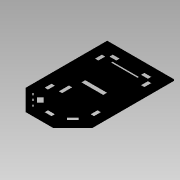
# Autodesk Inventor part: Base Kepala
Saved by Autodesk Inventor 2015 SP1 (Build 190203100, 203)
## iProperties
Created: 2015-02-13
Part Number: Base Kepala
Material: Generic
Document SubType Name: Modeling
Designer: Rafi Kurnia Putra
Density: 1 g/cm^3
Appearance: Default(1)
Author: Rafi Kurnia Putra
Autodesk Inventor part; units mm, degrees
ref_plane "YZ Plane" through (0, 0, 0) normal (1, 0, 0) x (0, 1, 0)
ref_plane "XZ Plane" through (0, 0, 0) normal (0, 1, 0) x (-1, 0, 0)
ref_plane "XY Plane" through (0, 0, 0) normal (0, 0, 1) x (1, 0, 0)
sketch "Sketch1" plane through (0, 0, 0) normal (0, 1, 0) x (-1, 0, 0)
  line L0 (31.6823, -78.8894) -> (44.0567, -66.5151)
  line L1 (24.6113, -71.8184) -> (31.6823, -78.8894)
  line L2 (36.9856, -59.444) -> (24.6113, -71.8184)
  line L3 (44.0567, -66.5151) -> (36.9856, -59.444)
  line L4 (8.75, -88.3884) -> (8.75, -78.3884)
  line L5 (-8.75, -88.3884) -> (8.75, -88.3884)
  line L6 (8.75, -78.3884) -> (-8.75, -78.3884)
  line L7 (-8.75, -78.3884) -> (-8.75, -88.3884)
  line L8 (-31.6827, -78.8894) -> (-24.6116, -71.8184)
  line L9 (-24.6116, -71.8184) -> (-36.986, -59.444)
  line L10 (-44.057, -66.5151) -> (-31.6827, -78.8894)
  line L11 (-36.986, -59.444) -> (-44.057, -66.5151)
  line L12 (-53.5557, -43.5826) -> (-43.5557, -43.5826)
  line L13 (-43.5557, -43.5826) -> (-43.5557, -26.0826)
  line L14 (-43.5557, -26.0826) -> (-53.5557, -26.0826)
  line L15 (-53.5557, -26.0826) -> (-53.5557, -43.5826)
  line L16 (-53.556, 80.1674) -> (-53.556, 62.6674)
  line L17 (-43.556, 80.1674) -> (-53.556, 80.1674)
  line L18 (-43.556, 62.6674) -> (-43.556, 80.1674)
  line L19 (-53.556, 62.6674) -> (-43.556, 62.6674)
  line L20 (-42.0848, 91.6386) -> (-42.0848, 81.6386)
  line L21 (-42.0848, 81.6386) -> (-24.5848, 81.6386)
  line L22 (-24.5848, 81.6386) -> (-24.5848, 91.6386)
  line L23 (-24.5848, 91.6386) -> (-42.0848, 91.6386)
  line L24 (42.0848, 91.6386) -> (24.5848, 91.6386)
  line L25 (42.0848, 81.6386) -> (42.0848, 91.6386)
  line L26 (24.5848, 81.6386) -> (42.0848, 81.6386)
  line L27 (24.5848, 91.6386) -> (24.5848, 81.6386)
  line L28 (43.556, 80.1674) -> (43.556, 62.6674)
  line L29 (53.556, 80.1674) -> (43.556, 80.1674)
  line L30 (53.556, 62.6674) -> (53.556, 80.1674)
  line L31 (43.556, 62.6674) -> (53.556, 62.6674)
  circle A0 centre (37.593, 75.6756) radius 1.75
  circle A1 centre (32.8575, 75.4371) radius 1.75
  circle A2 centre (50.5965, 88.6786) radius 1.75
  line L32 (29.3575, 78.4256) -> (-29.3575, 78.4256)
  line L33 (29.3575, 72.4486) -> (29.3575, 78.4256)
  line L34 (-29.3575, 72.4486) -> (29.3575, 72.4486)
  line L35 (-29.3575, 78.4256) -> (-29.3575, 72.4486)
  circle A3 centre (-32.8575, 75.4371) radius 1.75
  circle A4 centre (-37.593, 75.6756) radius 1.75
  circle A5 centre (-50.5965, 88.6786) radius 1.75
  line L36 (-24.5, 4.9331) -> (24.5, 4.9331)
  circle A6 centre (28, 4.9331) radius 1.75
  circle A7 centre (32.442, 26.7171) radius 1.5
  circle A8 centre (38, 31.4596) radius 1.75
  circle A9 centre (50.5965, 18.9376) radius 1.75
  circle A10 centre (32.4485, 53.6756) radius 1.75
  circle A11 centre (-32.4355, 53.6756) radius 1.75
  circle A12 centre (-50.5965, 18.9376) radius 1.75
  circle A13 centre (-32.442, 26.7171) radius 1.5
  circle A14 centre (-28, 4.9331) radius 1.75
  line L37 (-22.2, -10.9442) -> (-32, -10.9442)
  line L38 (-22.2, -35.1896) -> (-22.2, -10.9442)
  line L39 (-32, -35.1896) -> (-22.2, -35.1896)
  line L40 (-32, -10.9442) -> (-32, -35.1896)
  circle A15 centre (-49.906, -55.5042) radius 1.75
  circle A16 centre (-37.593, -48.9392) radius 1.75
  circle A17 centre (-20, -65.0669) radius 1.75
  circle A18 centre (13.2193, -19.3896) radius 1.75
  circle A19 centre (13.2193, -43.7996) radius 1.75
  circle A20 centre (20, -65.0669) radius 1.75
  circle A21 centre (37.593, -48.9392) radius 1.75
  circle A22 centre (39.7053, -43.7996) radius 1.75
  circle A23 centre (39.7053, -19.3896) radius 1.75
  circle A24 centre (49.9057, -55.5042) radius 1.75
  line L41 (43.5557, -43.5826) -> (53.5557, -43.5826)
  line L42 (43.5557, -26.0826) -> (43.5557, -43.5826)
  line L43 (53.5557, -26.0826) -> (43.5557, -26.0826)
  line L44 (53.5557, -43.5826) -> (53.5557, -26.0826)
  line L45 (24.5, 4.9331) -> (24.5, 15.9376)
  line L46 (24.5, 15.9376) -> (-24.5, 15.9376)
  line L47 (-24.5, 15.9376) -> (-24.5, 4.9331)
  circle A25 centre (14, 31.4596) radius 1.75
  circle A26 centre (-27.94, -53.8096) radius 1.75
  circle A27 centre (20.32, -47.4596) radius 1.75
  line L48 (70.4053, -63.9933) -> (29.1627, -105.2363)
  line L49 (29.1627, -105.2363) -> (-29.1634, -105.2362)
  line L50 (-29.1634, -105.2362) -> (-70.4063, -63.9936)
  line L51 (-70.4063, -63.9936) -> (-70.4063, 108.2408)
  line L52 (-70.4063, 108.2408) -> (70.4053, 108.2411)
  line L53 (70.4053, 108.2411) -> (70.4053, -63.9933)
  line L54 (37.7622, -79.6663) -> (44.8333, -72.5952)
  line L55 (44.8333, -72.5952) -> (46.2475, -74.0094)
  line L56 (46.2475, -74.0094) -> (39.1764, -81.0805)
  line L57 (39.1764, -81.0805) -> (37.7622, -79.6663)
  line L58 (37.7622, -79.6663) -> (46.2475, -74.0094) construction
  line L59 (44.8333, -72.5952) -> (39.1764, -81.0805) construction
  line L60 (34.2266, -83.2018) -> (27.1556, -90.2729)
  line L61 (27.1556, -90.2729) -> (28.5698, -91.6871)
  line L62 (28.5698, -91.6871) -> (35.6409, -84.616)
  line L63 (35.6409, -84.616) -> (34.2266, -83.2018)
  line L64 (34.2266, -83.2018) -> (28.5698, -91.6871) construction
  line L65 (27.1556, -90.2729) -> (35.6409, -84.616) construction
  line L66 (55.4401, -61.9888) -> (48.369, -69.0599)
  line L67 (48.369, -69.0599) -> (49.7828, -70.4737)
  line L68 (49.7828, -70.4737) -> (56.8539, -63.4026)
  line L69 (56.8539, -63.4026) -> (55.4401, -61.9888)
  line L70 (55.4401, -61.9888) -> (49.7828, -70.4737) construction
  line L71 (48.369, -69.0599) -> (56.8539, -63.4026) construction
  line L72 (5, -93.2363) -> (15, -93.2363) construction
  line L73 (-10, -93.2363) -> (-20, -93.2363)
  line L74 (-20, -93.2363) -> (-20, -95.2363)
  line L75 (-20, -95.2363) -> (-10, -95.2363)
  line L76 (-10, -95.2363) -> (-10, -93.2363)
  line L77 (-10, -93.2363) -> (-20, -95.2363) construction
  line L78 (-20, -93.2363) -> (-10, -95.2363) construction
  line L79 (-10, -93.2363) -> (0, -93.2363) construction
  line L80 (20, -95.2363) -> (10, -95.2363)
  line L81 (10, -95.2363) -> (10, -93.237)
  line L82 (10, -93.237) -> (20, -93.237)
  line L83 (20, -93.237) -> (20, -95.2363)
  line L84 (20, -95.2363) -> (10, -93.237) construction
  line L85 (10, -95.2363) -> (20, -93.237) construction
  line L86 (-7.5214, 96.2408) -> (7.4786, 96.2408)
  line L87 (7.4786, 96.2408) -> (7.4786, 98.2408)
  line L88 (7.4786, 98.2408) -> (-7.5214, 98.2408)
  line L89 (-7.5214, 98.2408) -> (-7.5214, 96.2408)
  line L90 (-7.5214, 96.2408) -> (7.4786, 98.2408) construction
  line L91 (7.4786, 96.2408) -> (-7.5214, 98.2408) construction
  line L92 (-7.5214, 96.2408) -> (7.4786, 96.2408) construction
  line L93 (60.4053, 25.443) -> (60.4053, 10.443)
  line L94 (60.4053, 10.443) -> (58.4053, 10.443)
  line L95 (58.4053, 10.443) -> (58.4053, 25.443)
  line L96 (58.4053, 25.443) -> (60.4053, 25.443)
  line L97 (60.4053, 25.443) -> (58.4053, 10.443) construction
  line L98 (60.4053, 10.443) -> (58.4053, 25.443) construction
  line L99 (-37.8487, -79.5805) -> (-44.9198, -72.5095)
  line L100 (-44.9198, -72.5095) -> (-46.334, -73.9237)
  line L101 (-46.334, -73.9237) -> (-39.2629, -80.9947)
  line L102 (-39.2629, -80.9947) -> (-37.8487, -79.5805)
  line L103 (-37.8487, -79.5805) -> (-46.334, -73.9237) construction
  line L104 (-34.3131, -83.116) -> (-27.242, -90.1871)
  line L105 (-27.242, -90.1871) -> (-28.6562, -91.6013)
  line L106 (-28.6562, -91.6013) -> (-35.7273, -84.5302)
  line L107 (-35.7273, -84.5302) -> (-34.3131, -83.116)
  line L108 (-34.3131, -83.116) -> (-28.6562, -91.6013) construction
  line L109 (-27.242, -90.1871) -> (-35.7273, -84.5302) construction
  line L110 (-55.5071, -61.8836) -> (-48.4359, -68.9546)
  line L111 (-48.4359, -68.9546) -> (-49.8695, -70.3882)
  line L112 (-49.8695, -70.3882) -> (-56.9406, -63.3172)
  line L113 (-56.9406, -63.3172) -> (-55.5071, -61.8836)
  line L114 (-55.5071, -61.8836) -> (-49.8695, -70.3882) construction
  line L115 (-48.4359, -68.9546) -> (-56.9406, -63.3172) construction
  line L116 (-60.4053, 25.443) -> (-60.4053, 10.443)
  line L117 (-60.4053, 10.443) -> (-58.4053, 10.443)
  line L118 (-58.4053, 10.443) -> (-58.4053, 25.443)
  line L119 (-58.4053, 25.443) -> (-60.4053, 25.443)
  line L120 (-60.4053, 25.443) -> (-58.4053, 10.443) construction
  line L121 (-60.4053, 10.443) -> (-58.4053, 25.443) construction
  line L122 (-58.4053, 42.943) -> (-58.4053, 57.943)
  line L123 (-58.4053, 57.943) -> (-60.4053, 57.943)
  line L124 (-60.4053, 57.943) -> (-60.4053, 42.943)
  line L125 (-60.4053, 57.943) -> (-58.4053, 42.943) construction
  line L126 (-60.4053, 42.943) -> (-58.4053, 57.943) construction
  line L127 (-60.4053, 42.943) -> (-58.4053, 42.943)
  line L128 (-58.4053, 75.443) -> (-58.4053, 90.443)
  line L129 (-58.4053, 90.443) -> (-60.4053, 90.443)
  line L130 (-60.4053, 90.443) -> (-60.4053, 75.443)
  line L131 (-60.4053, 90.443) -> (-58.4053, 75.443) construction
  line L132 (-60.4053, 75.443) -> (-58.4053, 90.443) construction
  line L133 (-60.4053, 75.443) -> (-58.4053, 75.443)
  line L134 (-58.4053, -22.057) -> (-58.4053, -7.057)
  line L135 (-58.4053, -7.057) -> (-60.4053, -7.057)
  line L136 (-60.4053, -7.057) -> (-60.4053, -22.057)
  line L137 (-60.4053, -7.057) -> (-58.4053, -22.057) construction
  line L138 (-60.4053, -22.057) -> (-58.4053, -7.057) construction
  line L139 (-60.4053, -22.057) -> (-58.4053, -22.057)
  line L140 (-58.4053, 10.443) -> (-58.4053, 25.443)
  line L141 (-58.4053, 25.443) -> (-60.4053, 25.443)
  line L142 (-60.4053, 25.443) -> (-60.4053, 10.443)
  line L143 (-60.4053, 25.443) -> (-58.4053, 10.443) construction
  line L144 (-60.4053, 10.443) -> (-58.4053, 25.443) construction
  line L145 (-60.4053, 10.443) -> (-58.4053, 10.443)
  line L146 (-58.4053, 42.943) -> (-58.4053, 57.943)
  line L147 (-58.4053, 57.943) -> (-60.4053, 57.943)
  line L148 (-60.4053, 57.943) -> (-60.4053, 42.943)
  line L149 (-60.4053, 57.943) -> (-58.4053, 42.943) construction
  line L150 (-60.4053, 42.943) -> (-58.4053, 57.943) construction
  line L151 (-60.4053, 42.943) -> (-58.4053, 42.943)
  line L152 (-58.4063, -54.3943) -> (-58.4063, -39.3943)
  line L153 (-58.4063, -39.3943) -> (-60.4063, -39.3943)
  line L154 (-60.4063, -39.3943) -> (-60.4063, -54.3943)
  line L155 (-60.4063, -39.3943) -> (-58.4063, -54.3943) construction
  line L156 (-60.4063, -54.3943) -> (-58.4063, -39.3943) construction
  line L157 (-60.4063, -54.3943) -> (-58.4063, -54.3943)
  line L158 (-58.4063, -21.8943) -> (-58.4063, -6.8943)
  line L159 (-58.4063, -6.8943) -> (-60.4063, -6.8943)
  line L160 (-60.4063, -6.8943) -> (-60.4063, -21.8943)
  line L161 (-60.4063, -6.8943) -> (-58.4063, -21.8943) construction
  line L162 (-60.4063, -21.8943) -> (-58.4063, -6.8943) construction
  line L163 (-60.4063, -21.8943) -> (-58.4063, -21.8943)
  line L164 (-58.4053, 10.443) -> (-58.4053, 25.443)
  line L165 (-58.4053, 25.443) -> (-60.4053, 25.443)
  line L166 (-60.4053, 25.443) -> (-60.4053, 10.443)
  line L167 (-60.4053, 25.443) -> (-58.4053, 10.443) construction
  line L168 (-60.4053, 10.443) -> (-58.4053, 25.443) construction
  line L169 (-60.4053, 10.443) -> (-58.4053, 10.443)
  line L170 (15.4786, 96.2409) -> (30.4786, 96.2409)
  line L171 (30.4786, 96.2409) -> (30.4786, 98.2409)
  line L172 (30.4786, 98.2409) -> (15.4786, 98.2409)
  line L173 (15.4786, 98.2409) -> (15.4786, 96.2409)
  line L174 (15.4786, 96.2409) -> (30.4786, 98.2409) construction
  line L175 (30.4786, 96.2409) -> (15.4786, 98.2409) construction
  line L176 (15.4786, 96.2409) -> (30.4786, 96.2409) construction
  line L177 (38.4786, 96.2409) -> (53.4786, 96.2409)
  line L178 (53.4786, 96.2409) -> (53.4786, 98.2409)
  line L179 (53.4786, 98.2409) -> (38.4786, 98.2409)
  line L180 (38.4786, 98.2409) -> (38.4786, 96.2409)
  line L181 (38.4786, 96.2409) -> (53.4786, 98.2409) construction
  line L182 (53.4786, 96.2409) -> (38.4786, 98.2409) construction
  line L183 (38.4786, 96.2409) -> (53.4786, 96.2409) construction
  line L184 (-30.5214, 96.2408) -> (-15.5214, 96.2408)
  line L185 (-15.5214, 96.2408) -> (-15.5214, 98.2408)
  line L186 (-15.5214, 98.2408) -> (-30.5214, 98.2408)
  line L187 (-30.5214, 98.2408) -> (-30.5214, 96.2408)
  line L188 (-30.5214, 96.2408) -> (-15.5214, 98.2408) construction
  line L189 (-15.5214, 96.2408) -> (-30.5214, 98.2408) construction
  line L190 (-30.5214, 96.2408) -> (-15.5214, 96.2408) construction
  line L191 (-7.5214, 96.2408) -> (7.4786, 96.2408)
  line L192 (7.4786, 96.2408) -> (7.4786, 98.2408)
  line L193 (7.4786, 98.2408) -> (-7.5214, 98.2408)
  line L194 (-7.5214, 98.2408) -> (-7.5214, 96.2408)
  line L195 (-7.5214, 96.2408) -> (7.4786, 98.2408) construction
  line L196 (7.4786, 96.2408) -> (-7.5214, 98.2408) construction
  line L197 (-7.5214, 96.2408) -> (7.4786, 96.2408) construction
  line L198 (15.4786, 96.2409) -> (30.4786, 96.2409)
  line L199 (30.4786, 96.2409) -> (30.4786, 98.2409)
  line L200 (30.4786, 98.2409) -> (15.4786, 98.2409)
  line L201 (15.4786, 98.2409) -> (15.4786, 96.2409)
  line L202 (15.4786, 96.2409) -> (30.4786, 98.2409) construction
  line L203 (30.4786, 96.2409) -> (15.4786, 98.2409) construction
  line L204 (15.4786, 96.2409) -> (30.4786, 96.2409) construction
  line L205 (-53.5214, 96.2407) -> (-38.5214, 96.2407)
  line L206 (-38.5214, 96.2407) -> (-38.5214, 98.2407)
  line L207 (-38.5214, 98.2407) -> (-53.5214, 98.2407)
  line L208 (-53.5214, 98.2407) -> (-53.5214, 96.2407)
  line L209 (-53.5214, 96.2407) -> (-38.5214, 98.2407) construction
  line L210 (-38.5214, 96.2407) -> (-53.5214, 98.2407) construction
  line L211 (-53.5214, 96.2407) -> (-38.5214, 96.2407) construction
  line L212 (-30.5214, 96.2408) -> (-15.5214, 96.2408)
  line L213 (-15.5214, 96.2408) -> (-15.5214, 98.2408)
  line L214 (-15.5214, 98.2408) -> (-30.5214, 98.2408)
  line L215 (-30.5214, 98.2408) -> (-30.5214, 96.2408)
  line L216 (-30.5214, 96.2408) -> (-15.5214, 98.2408) construction
  line L217 (-15.5214, 96.2408) -> (-30.5214, 98.2408) construction
  line L218 (-30.5214, 96.2408) -> (-15.5214, 96.2408) construction
  line L219 (-7.5214, 96.2408) -> (7.4786, 96.2408)
  line L220 (7.4786, 96.2408) -> (7.4786, 98.2408)
  line L221 (7.4786, 98.2408) -> (-7.5214, 98.2408)
  line L222 (-7.5214, 98.2408) -> (-7.5214, 96.2408)
  line L223 (-7.5214, 96.2408) -> (7.4786, 98.2408) construction
  line L224 (7.4786, 96.2408) -> (-7.5214, 98.2408) construction
  line L225 (-7.5214, 96.2408) -> (7.4786, 96.2408) construction
  line L226 (60.4053, 57.943) -> (60.4053, 42.943)
  line L227 (60.4053, 42.943) -> (58.4053, 42.943)
  line L228 (58.4053, 42.943) -> (58.4053, 57.943)
  line L229 (58.4053, 57.943) -> (60.4053, 57.943)
  line L230 (60.4053, 57.943) -> (58.4053, 42.943) construction
  line L231 (60.4053, 42.943) -> (58.4053, 57.943) construction
  line L232 (60.4053, 90.443) -> (60.4053, 75.443)
  line L233 (60.4053, 75.443) -> (58.4053, 75.443)
  line L234 (58.4053, 75.443) -> (58.4053, 90.443)
  line L235 (58.4053, 90.443) -> (60.4053, 90.443)
  line L236 (60.4053, 90.443) -> (58.4053, 75.443) construction
  line L237 (60.4053, 75.443) -> (58.4053, 90.443) construction
  line L238 (60.4053, -7.057) -> (60.4053, -22.057)
  line L239 (60.4053, -22.057) -> (58.4053, -22.057)
  line L240 (58.4053, -22.057) -> (58.4053, -7.057)
  line L241 (58.4053, -7.057) -> (60.4053, -7.057)
  line L242 (60.4053, -7.057) -> (58.4053, -22.057) construction
  line L243 (60.4053, -22.057) -> (58.4053, -7.057) construction
  line L244 (60.4053, 25.443) -> (60.4053, 10.443)
  line L245 (60.4053, 10.443) -> (58.4053, 10.443)
  line L246 (58.4053, 10.443) -> (58.4053, 25.443)
  line L247 (58.4053, 25.443) -> (60.4053, 25.443)
  line L248 (60.4053, 25.443) -> (58.4053, 10.443) construction
  line L249 (60.4053, 10.443) -> (58.4053, 25.443) construction
  line L250 (60.4053, 57.943) -> (60.4053, 42.943)
  line L251 (60.4053, 42.943) -> (58.4053, 42.943)
  line L252 (58.4053, 42.943) -> (58.4053, 57.943)
  line L253 (58.4053, 57.943) -> (60.4053, 57.943)
  line L254 (60.4053, 57.943) -> (58.4053, 42.943) construction
  line L255 (60.4053, 42.943) -> (58.4053, 57.943) construction
  line L256 (60.4053, -39.557) -> (60.4053, -54.557)
  line L257 (60.4053, -54.557) -> (58.4053, -54.557)
  line L258 (58.4053, -54.557) -> (58.4053, -39.557)
  line L259 (58.4053, -39.557) -> (60.4053, -39.557)
  line L260 (60.4053, -39.557) -> (58.4053, -54.557) construction
  line L261 (60.4053, -54.557) -> (58.4053, -39.557) construction
  line L262 (60.4053, -7.057) -> (60.4053, -22.057)
  line L263 (60.4053, -22.057) -> (58.4053, -22.057)
  line L264 (58.4053, -22.057) -> (58.4053, -7.057)
  line L265 (58.4053, -7.057) -> (60.4053, -7.057)
  line L266 (60.4053, -7.057) -> (58.4053, -22.057) construction
  line L267 (60.4053, -22.057) -> (58.4053, -7.057) construction
  line L268 (60.4053, 25.443) -> (60.4053, 10.443)
  line L269 (60.4053, 10.443) -> (58.4053, 10.443)
  line L270 (58.4053, 10.443) -> (58.4053, 25.443)
  line L271 (58.4053, 25.443) -> (60.4053, 25.443)
  line L272 (60.4053, 25.443) -> (58.4053, 10.443) construction
  line L273 (60.4053, 10.443) -> (58.4053, 25.443) construction
  point P0 (0, 0)
  point P1 (42.0048, -76.8379)
  point P2 (31.3982, -87.4444)
  point P3 (52.6114, -66.2313)
  point P4 (-15, -94.2363)
  point P5 (15, -94.2366)
  point P6 (-0.0214, 97.2408)
  point P7 (59.4053, 17.943)
  point P8 (-31.4847, -87.3586)
  point P9 (-52.6883, -66.1359)
  point P10 (-65.5064, -62.0457)
  point P11 (-59.4053, 17.943)
  point P12 (-59.4053, 50.443)
  point P13 (-59.4053, 82.943)
  point P14 (-59.4053, -14.557)
  point P15 (-59.4053, 17.943)
  point P16 (-59.4053, 50.443)
  point P17 (-59.4063, -46.8943)
  point P18 (-59.4063, -14.3943)
  point P19 (-59.4053, 17.943)
  point P20 (22.9786, 97.2409)
  point P21 (45.9786, 97.2409)
  point P22 (-23.0214, 97.2408)
  point P23 (-0.0214, 97.2408)
  point P24 (22.9786, 97.2409)
  point P25 (-46.0214, 97.2407)
  point P26 (-23.0214, 97.2408)
  point P27 (-0.0214, 97.2408)
  point P28 (59.4053, 50.443)
  point P29 (59.4053, 82.943)
  point P30 (59.4053, -14.557)
  point P31 (59.4053, 17.943)
  point P32 (59.4053, 50.443)
  point P33 (59.4053, -47.057)
  point P34 (59.4053, -14.557)
  point P35 (59.4053, 17.943)
  dimension "d106" = 23
  dimension "d109" = 23
  dimension "d115" = 32.5
  dimension "d118" = 32.5
  dimension "d121" = 172.2345
  dimension "d122" = 140.8117
  dimension "d123" = 172.2345
  dimension "d124" = 58.3261
  dimension "d125" = 58.3261
  dimension "d126" = 58.3261
  dimension "d127" = 135
  dimension "d128" = 135
  dimension "d129" = 135
  dimension "d130" = 135
  dimension "d131" = 90
  dimension "d132" = 90
  dimension "d134" = 10
  dimension "d135" = 9.9999
  dimension "d136" = 10
  dimension "d137" = 10
  dimension "d138" = 10
  dimension "d145" = 80.298
  constraints: 548 end point, 68 midpoint, 28 centre point, 14 parallel, 8 collinear, 7 perpendicular, 6 horizontal, 3 vertical, 194 other
  measures "d106" distance of L87.end L171.end
  measures "d109" distance of L87.end L185.end
  measures "d115" distance of L94.end L228.start
  measures "d118" distance of L94.end L240.start
  measures "d121" distance of L52.end L48.start
  measures "d122" distance of L51.end L52.end
  measures "d123" distance of L50.end L51.end
  measures "d124" distance of L48.end L49.end
  measures "d125" distance of L48.start L48.end
  measures "d126" distance of L49.end L50.end
  measures "d127" angle of L48 L53
  measures "d128" angle of L49 L48
  measures "d129" angle of L49 L50
  measures "d130" angle of L50 L51
  measures "d131" angle of L52 L51
  measures "d132" angle of L53 L52
  measures "d134" distance from line of L48.end L80
  measures "d135" distance from line of L49.end L75
  measures "d136" distance from line of L49.end L106
  measures "d137" distance from line of L50.end L112
  measures "d138" distance from line of L49.end L101
  measures "d145" distance from line of point (59.405, 17.943) L179
extrude "Extrusion2" add sketch "Sketch1" along normal blind 3
body "Solid2"
